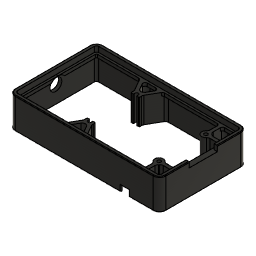
Apollo Vmount Body P3 [(P)MPLA000000170] v1 (Autodesk Fusion 360 design; units mm, degrees)
Autodesk Fusion 360 part; units mm, degrees
sketch "Sketch1" plane through (0, 0, 0) normal (0, 0, 1) x (1, 0, 0)
  line L0 (-70.75, 35.15) -> (-70.75, -35.15)
  arc A0 (-70.75, -35.15) -> (-64.75, -41.15) centre (-64.75, -35.15) ccw
  line L1 (-64.75, -41.15) -> (64.75, -41.15)
  arc A1 (64.75, -41.15) -> (70.75, -35.15) centre (64.75, -35.15) ccw
  line L2 (70.75, -35.15) -> (70.75, 35.15)
  arc A2 (70.75, 35.15) -> (64.75, 41.15) centre (64.75, 35.15) ccw
  line L3 (64.75, 41.15) -> (-64.75, 41.15)
  arc A3 (-64.75, 41.15) -> (-70.75, 35.15) centre (-64.75, 35.15) ccw
  circle A4 centre (-14, 22.05) radius 1.6
  circle A5 centre (51.15, -21.95) radius 4
  circle A6 centre (51.15, 22.05) radius 4
  line L4 (-14, -21.95) -> (70.75, -21.95)
  line L5 (-14, 41.15) -> (-14, -46.1385)
  line L6 (-14, 22.05) -> (87.0646, 22.05)
  circle A7 centre (-14, -21.95) radius 1.6
  line L7 (-15.5, 41.15) -> (-15.5, -46.1385)
  line L8 (-12.5, 41.15) -> (-12.5, -46.1385)
  line L9 (-65.75, -38.15) -> (65.75, -38.15)
  arc A8 (65.75, -38.15) -> (67.75, -36.15) centre (65.75, -36.15) ccw
  line L10 (67.75, -36.15) -> (67.75, 36.15)
  arc A9 (67.75, 36.15) -> (65.75, 38.15) centre (65.75, 36.15) ccw
  line L11 (65.75, 38.15) -> (-65.75, 38.15)
  arc A10 (-65.75, 38.15) -> (-67.75, 36.15) centre (-65.75, 36.15) ccw
  line L12 (-67.75, 36.15) -> (-67.75, -36.15)
  arc A11 (-67.75, -36.15) -> (-65.75, -38.15) centre (-65.75, -36.15) ccw
  line L13 (51.15, -41.15) -> (51.15, 41.15)
  line L14 (52.65, -41.15) -> (52.65, 41.15)
  line L15 (49.65, -41.15) -> (49.65, 41.15)
  line L16 (-14, -23.45) -> (70.75, -23.45)
  line L17 (-17.7081, -20.45) -> (70.75, -20.45)
  line L18 (-17.7081, 20.55) -> (87.0646, 20.55)
  line L19 (-14, 23.55) -> (87.0646, 23.55)
  circle A12 centre (-14, -21.95) radius 4
  circle A13 centre (-14, 22.05) radius 4
  line L20 (-15.5, 25.7581) -> (-22.6545, 38.15)
  line L21 (-15.5, -25.6581) -> (-22.7122, -38.15)
  line L22 (-17.7003, -23.4691) -> (-26.1763, -38.15)
  line L23 (-17.7003, 23.5691) -> (-26.1186, 38.15)
  line L24 (-12.5, 25.7581) -> (-5.3455, 38.15)
  line L25 (-12.5, -25.6581) -> (-5.2878, -38.15)
  line L26 (-10.3107, -23.45) -> (-1.8237, -38.15)
  line L27 (-10.2997, 23.5691) -> (-1.8814, 38.15)
  circle A14 centre (51.15, -21.95) radius 1.6
  circle A15 centre (51.15, 22.05) radius 1.6
  line L28 (-15, 41.15) -> (-15, -46.1385)
  line L29 (-13, 41.15) -> (-13, -46.1385)
  dimension "d49" = 3.2
  dimension "d50" = 8
  dimension "d51" = 8
  dimension "d52" = 6
  dimension "d53" = 82.3
  dimension "d54" = 41.15
  dimension "d55" = 141.5
  dimension "d56" = 70.75
  dimension "d57" = 3.2
  dimension "d58" = 19.6
  dimension "d59" = 19.2
  dimension "d60" = 65.15
  dimension "d61" = 44
  dimension "d62" = 1.5
  dimension "d63" = -1.5
  dimension "d65" = 1.5
  dimension "d66" = -1.5
  dimension "d67" = 1.5
  dimension "d71" = -1.5
  dimension "d72" = 8
  dimension "d73" = 8
  dimension "d74" = 60
  dimension "d75" = 60
  dimension "d78" = 3
  dimension "d79" = 3
  dimension "d80" = 60
  dimension "d81" = 60
  dimension "d84" = 3
  dimension "d85" = 3
  dimension "d86" = 3.2
  dimension "d87" = 3.2
  dimension "d107" = 1
  dimension "d108" = -1
  dimension "d111" = 2
  dimension "d112" = 2
  dimension "d113" = 6
  dimension "d114" = 6
  dimension "d115" = 6
  constraint horizontal L3
  constraint perpendicular L0 L3
  constraint parallel L1 L3
  constraint parallel L0 L2
  constraint tangent L3 A3
  constraint tangent L0 A3
  constraint tangent L0 A0
  constraint tangent A0 L1
  constraint tangent L1 A1
  constraint tangent A1 L2
  constraint tangent L2 A2
  constraint tangent A2 L3
  constraint perpendicular L1 L5
  constraint coincident A4.centre L6.start
  constraint perpendicular L2 L6
  constraint coincident L2 L4.end
  constraint coincident L3 L5.start
  constraint coincident L4.start L5
  constraint perpendicular L4 L5
  constraint coincident L4.start A7.centre
  constraint vertical A5.centre A6.centre
  constraint coincident A5.centre L4
  constraint vertical A4.centre L4.start
  constraint coincident A6.centre L6
  constraint coincident L1 L13.start
  constraint coincident L3 L13.end
  constraint coincident A5.centre L13
  constraint coincident A6.centre L13
  constraint concentric A7 A12
  constraint concentric A4 A13
  constraint coincident A13 L20.start
  constraint coincident L7 L20.start
  constraint coincident L11 L20.end
  constraint coincident A12 L21.start
  constraint coincident L7 L21.start
  constraint coincident L9 L21.end
  constraint parallel L21 L22
  constraint coincident A12 L22.start
  constraint coincident L9 L22.end
  constraint parallel L20 L23
  constraint coincident A13 L23.start
  constraint coincident L11 L23.end
  constraint coincident A13 L24.start
  constraint coincident L8 L24.start
  constraint coincident L11 L24.end
  constraint coincident A12 L25.start
  constraint coincident L9 L25.end
  constraint parallel L25 L26
  constraint coincident L9 L26.end
  constraint coincident L16 L26.start
  constraint parallel L24 L27
  constraint coincident A13 L27.start
  constraint coincident L11 L27.end
  constraint coincident L8 L25.start
  constraint concentric A5 A14
  constraint concentric A6 A15
  constraint parallel L4 L17
  constraint coincident A12 L17.start
  constraint parallel L6 L18
  constraint coincident A13 L18.start
  constraint parallel L1 L9
  constraint parallel L2 L10
  constraint parallel L3 L11
  constraint parallel L0 L12
  constraint tangent A9 L11
  constraint tangent L9 A11
  constraint tangent L9 A8
  constraint tangent A10 L12
  constraint tangent A8 L10
  constraint tangent L10 A9
  constraint tangent L12 A11
  constraint tangent L11 A10
  measures "d49" diameter of A4
  measures "d50" diameter of A6
  measures "d51" diameter of A5
  measures "d52" radius of A3
  measures "d53" distance of L1 L3
  measures "d54" distance of origin L1
  measures "d55" distance of L0 L2
  measures "d56" distance of origin L2
  measures "d57" diameter of A7
  measures "d58" distance of A5.centre L2
  measures "d59" distance of A5.centre L1
  measures "d60" distance of A5.centre L4.start
  measures "d61" distance of A5.centre A6.centre
  measures "d72" diameter of A12
  measures "d73" diameter of A13
  measures "d74" angle of L9 L21
  measures "d75" angle of L11 L20
  measures "d78" distance of L21 L22
  measures "d79" distance of L20 L23
  measures "d80" angle of L9 L25
  measures "d81" angle of L11 L24
  measures "d84" distance of L25 L26
  measures "d85" distance of L24 L27
  measures "d86" diameter of A14
  measures "d87" diameter of A15
  measures "d111" radius of A10
  measures "d112" radius of A11
  measures "d113" radius of A0
  measures "d114" radius of A1
  measures "d115" radius of A2
extrude "Extrude1" add sketch "Sketch1" along normal blind 29 contours L0 A0 L1 L3 A3 L7 L9 L11 A10 L12 A11 | L3 L7 L11 L28 | L1 L7 L9 L28 | L3 L5 L11 L28 | L1 L5 L9 L28 | L3 L5 L11 L29 | A4 L7 A13 L28 | A4 L7 L18 A13 | L11 A13 L20 L23 | L1 L5 L9 L29 | A7 L7 L17 A12 | L9 A12 L21 L22 | A7 L7 A12 L28 | L3 L8 L11 L29 | A4 L5 A13 L28 | L1 L8 L9 L29 | L5 A7 A12 L28 | L3 L8 L11 L15 | A4 L5 L19 A13 L29 | A4 L7 L18 L28 | L1 L8 L9 L15 | L5 A7 L16 A12 L29 | A7 L7 L17 L28 | L3 L11 L13 L15 | L8 L19 A13 L29 | L1 L9 L13 L15 | L8 L16 A12 L29 | L3 L11 L13 L14 | A6 L11 L13 L15 | L8 L19 A13 | L11 A13 L24 L27 | A4 L19 L29 | A4 L8 L19 L29 | L1 L9 L13 L14 | A5 L9 L13 L15 | L8 L16 A12 L26 | L9 A12 L25 L26 | A7 L8 L16 L29 | A7 L16 L29 | L2 A2 L3 L10 A9 L11 L14 L19 | A6 L11 L13 L14 | A6 L15 L19 | A6 L13 L15 L19 A15 | A4 L6 L8 L19 A13 | L1 A1 L2 L9 A8 L10 L14 L16 | A5 L9 L13 L14 | A5 L13 L15 L16 A14 | A5 L15 L16 | L4 A7 L8 L16 A12 | L16 A12 L26 | A6 L13 L14 L19 A15 | A6 L6 L15 L19 A15 | L15 L19 A15 | A5 L13 L14 L16 A14 | A5 L4 L15 L16 A14 | L15 L16 A14 | A6 L14 L19 | A6 L6 L15 L18 A15 | A4 L6 L8 L18 A13 | A4 L8 L18 L29 | A5 L14 L16 | A5 L4 L15 L17 A14 | L4 A7 L8 L17 A12 | A7 L8 L17 L29 | L2 L6 L10 L19 | A6 L6 L10 L19 | A6 L6 L14 L19 A15 | L14 L19 A15 | A6 L15 L18 | L2 L4 L10 L16 | A5 L4 L14 L16 A14 | A5 L4 L10 L16 | L14 L16 A14 | A5 L15 L17 | L2 L6 L10 L18 | A6 L6 L10 L18 | A6 L6 L14 L18 A15 | A6 L13 L15 L18 A15 | L15 L18 A15 | L2 L4 L10 L17 | A5 L4 L14 L17 A14 | A5 L4 L10 L17 | A5 L13 L15 L17 A14 | L15 L17 A14 | L2 L10 L17 L18 | A6 L14 L18 | A6 L13 L14 L18 A15 | A5 L14 L17 | A5 L13 L14 L17 A14 | L14 L18 A15 | L14 L17 A14
fillet "Fillet1" radius 3 32 edges at (-1.8237, -38.15, 14.5) (-22.7122, -38.15, 14.5) (-5.2878, -38.15, 14.5) (-26.1763, -38.15, 14.5) (-17.7003, -23.4691, 14.5) (-15.5, -25.6581, 14.5) (-12.5, -25.6581, 14.5) (54.8581, -20.45, 14.5) (54.8581, -23.45, 14.5) (52.65, -25.6581, 14.5) (49.65, -25.6581, 14.5) (52.65, -38.15, 14.5) (49.65, -38.15, 14.5) (67.75, -23.45, 14.5) (67.75, -20.45, 14.5) (-15.5, 25.7581, 14.5) (-12.5, 25.7581, 14.5) (-10.2997, 23.5691, 14.5) (-17.7003, 23.5691, 14.5) (-26.1186, 38.15, 14.5) (-22.6545, 38.15, 14.5) (-5.3455, 38.15, 14.5) (-1.8814, 38.15, 14.5) (49.65, 38.15, 14.5) (52.65, 38.15, 14.5) (52.65, 25.7581, 14.5) (54.8581, 23.55, 14.5) (49.65, 25.7581, 14.5) (67.75, 20.55, 14.5) (67.75, 23.55, 14.5) (54.8581, 20.55, 14.5) (-10.2997, -23.4691, 14.5)
sketch "Sketch2" plane through (0, 0, 29) normal (0, 0, 1) x (-1, 0, 0)
  arc A0 (-48.5786, -25.1139) -> (-54.2139, -19.4786) centre (-51.15, -22.05) ccw
  line L0 (-52.65, -27.4119) -> (-52.65, -35.15)
  line L1 (17.4583, -38.15) -> (10.5417, -38.15)
  arc A1 (-67.75, -36.15) -> (-65.75, -38.15) centre (-64.75, -35.15) ccw
  line L2 (-67.75, -17.55) -> (-67.75, 17.45)
  arc A2 (-65.75, 38.15) -> (-67.75, 36.15) centre (-64.75, 35.15) ccw
  line L3 (-65.75, 38.15) -> (-55.65, 38.15)
  line L4 (-52.65, 35.15) -> (-52.65, 27.3119)
  arc A3 (-54.2139, 19.3786) -> (-48.5786, 25.0139) centre (-51.15, 21.95) ccw
  line L5 (-49.65, 27.3119) -> (-49.65, 35.15)
  line L6 (-46.65, 38.15) -> (0.0916, 38.15)
  arc A4 (67.75, 36.15) -> (65.75, 38.15) centre (64.75, 35.15) ccw
  line L7 (67.75, 36.15) -> (67.75, -36.15)
  arc A5 (65.75, -38.15) -> (67.75, -36.15) centre (64.75, -35.15) ccw
  line L8 (65.75, -38.15) -> (27.8506, -38.15)
  line L9 (-49.65, -35.15) -> (-49.65, -27.4119)
  arc A6 (64.75, -41.15) -> (70.75, -35.15) centre (64.75, -35.15) ccw
  line L10 (70.75, -35.15) -> (70.75, 35.15)
  arc A7 (70.75, 35.15) -> (64.75, 41.15) centre (64.75, 35.15) ccw
  line L11 (64.75, 41.15) -> (-64.75, 41.15)
  arc A8 (-64.75, 41.15) -> (-70.75, 35.15) centre (-64.75, 35.15) ccw
  line L12 (-70.75, 35.15) -> (-70.75, -35.15)
  arc A9 (-70.75, -35.15) -> (-64.75, -41.15) centre (-64.75, -35.15) ccw
  line L13 (-64.75, -41.15) -> (64.75, -41.15)
  line L14 (25.2525, -36.65) -> (18.317, -24.6372)
  arc A10 (10.2919, -20.55) -> (10.0485, -22.6713) centre (14, -22.05) ccw
  line L15 (9.683, -24.6372) -> (2.7475, -36.65)
  line L16 (-64.75, -23.55) -> (-56.5119, -23.55)
  line L17 (13, -20.55) -> (10.2919, -20.55)
  line L18 (-64.75, 20.45) -> (-56.5119, 20.45)
  line L19 (-56.5119, 23.45) -> (-64.75, 23.45)
  line L20 (2.6897, 36.65) -> (9.683, 24.5372)
  arc A11 (10.0485, 22.5713) -> (10.2919, 20.45) centre (14, 21.95) ccw
  line L21 (18.317, 24.5372) -> (25.3103, 36.65)
  line L22 (20.1141, 33.65) -> (16.5981, 27.56)
  line L23 (11.4019, 27.56) -> (7.8859, 33.65)
  line L24 (16.5981, -27.66) -> (20.0564, -33.65)
  line L25 (7.9436, -33.65) -> (11.4019, -27.66)
  circle A12 centre (-51.15, 21.95) radius 1.6
  circle A13 centre (-51.15, -22.05) radius 1.6
  arc A14 (7.9436, -33.65) -> (10.5417, -38.15) centre (10.5417, -35.15) ccw
  arc A15 (16.5981, -27.66) -> (11.4019, -27.66) centre (14, -29.16) ccw
  arc A16 (17.4583, -38.15) -> (20.0564, -33.65) centre (17.4583, -35.15) ccw
  arc A17 (-49.65, 27.3119) -> (-48.5786, 25.0139) centre (-46.65, 27.3119) ccw
  arc A18 (-46.65, 38.15) -> (-49.65, 35.15) centre (-46.65, 35.15) ccw
  arc A19 (2.6897, 36.65) -> (0.0916, 38.15) centre (0.0916, 35.15) ccw
  arc A20 (18.317, 24.5372) -> (17.9515, 22.5713) centre (20.915, 23.0372) ccw
  arc A21 (27.9084, 38.15) -> (25.3103, 36.65) centre (27.9084, 35.15) ccw
  line L26 (27.9084, 38.15) -> (65.75, 38.15)
  arc A22 (25.2525, -36.65) -> (27.8506, -38.15) centre (27.8506, -35.15) ccw
  arc A23 (17.9515, -22.6713) -> (18.317, -24.6372) centre (20.915, -23.1372) ccw
  arc A24 (9.683, -24.6372) -> (10.0485, -22.6713) centre (7.085, -23.1372) ccw
  arc A25 (0.1494, -38.15) -> (2.7475, -36.65) centre (0.1494, -35.15) ccw
  line L27 (0.1494, -38.15) -> (-46.65, -38.15)
  arc A26 (-49.65, -35.15) -> (-46.65, -38.15) centre (-46.65, -35.15) ccw
  arc A27 (-48.5786, -25.1139) -> (-49.65, -27.4119) centre (-46.65, -27.4119) ccw
  arc A28 (-56.5119, -20.55) -> (-54.2139, -19.4786) centre (-56.5119, -17.55) ccw
  arc A29 (-67.75, -17.55) -> (-64.75, -20.55) centre (-64.75, -17.55) ccw
  arc A30 (-64.75, 20.45) -> (-67.75, 17.45) centre (-64.75, 17.45) ccw
  arc A31 (-54.2139, 19.3786) -> (-56.5119, 20.45) centre (-56.5119, 17.45) ccw
  arc A32 (-53.7214, 25.0139) -> (-52.65, 27.3119) centre (-55.65, 27.3119) ccw
  arc A33 (-53.7214, 25.0139) -> (-54.2139, 24.5214) centre (-51.15, 21.95) ccw
  arc A34 (-56.5119, 23.45) -> (-54.2139, 24.5214) centre (-56.5119, 26.45) ccw
  arc A35 (-67.75, 26.45) -> (-64.75, 23.45) centre (-64.75, 26.45) ccw
  line L28 (-67.75, 26.45) -> (-67.75, 36.15)
  arc A36 (-52.65, 35.15) -> (-55.65, 38.15) centre (-55.65, 35.15) ccw
  arc A37 (-55.65, -38.15) -> (-52.65, -35.15) centre (-55.65, -35.15) ccw
  line L29 (-55.65, -38.15) -> (-65.75, -38.15)
  line L30 (-67.75, -36.15) -> (-67.75, -26.55)
  arc A38 (-64.75, -23.55) -> (-67.75, -26.55) centre (-64.75, -26.55) ccw
  arc A39 (-54.2139, -24.6214) -> (-56.5119, -23.55) centre (-56.5119, -26.55) ccw
  arc A40 (-54.2139, -24.6214) -> (-53.7214, -25.1139) centre (-51.15, -22.05) ccw
  arc A41 (-52.65, -27.4119) -> (-53.7214, -25.1139) centre (-55.65, -27.4119) ccw
  arc A42 (11.4019, 27.56) -> (16.5981, 27.56) centre (14, 29.06) ccw
  arc A43 (10.0485, 22.5713) -> (9.683, 24.5372) centre (7.085, 23.0372) ccw
  line L31 (27.8506, -38.15) -> (-55.65, -38.15)
  line L32 (-67.75, -36.15) -> (-67.75, 26.45)
  line L33 (-55.65, 38.15) -> (27.9084, 38.15)
  line L34 (-67.75, 13.2) -> (-70.75, 13.2)
  line L35 (-67.75, -13.2) -> (-70.75, -13.2)
  arc A44 (13, -20.801) -> (15, -20.801) centre (14, -22.05) ccw
  line L36 (-56.5119, -20.55) -> (-64.75, -20.55)
  line L37 (10.2919, 20.45) -> (13, 20.45)
  arc A45 (15, 20.701) -> (13, 20.701) centre (14, 21.95) ccw
  arc A46 (17.7081, 20.45) -> (17.9515, 22.5713) centre (14, 21.95) ccw
  arc A47 (17.9515, -22.6713) -> (17.7081, -20.55) centre (14, -22.05) ccw
  line L38 (17.7081, -20.55) -> (15, -20.55)
  arc A48 (10.484, 38.15) -> (7.8859, 33.65) centre (10.484, 35.15) ccw
  line L39 (10.484, 38.15) -> (17.516, 38.15)
  arc A49 (20.1141, 33.65) -> (17.516, 38.15) centre (17.516, 35.15) ccw
  line L40 (13, 20.45) -> (13, 20.701)
  line L41 (15, 20.701) -> (15, 20.45)
  line L42 (15, 20.45) -> (17.7081, 20.45)
  line L43 (15, -20.55) -> (15, -20.801)
  line L44 (13, -20.801) -> (13, -20.55)
  line L45 (65.75, -35.15) -> (65.75, 35.15)
  arc A50 (65.75, 35.15) -> (64.75, 36.15) centre (64.75, 35.15) ccw
  line L46 (64.75, 36.15) -> (-64.75, 36.15)
  arc A51 (-64.75, 36.15) -> (-65.75, 35.15) centre (-64.75, 35.15) ccw
  line L47 (-65.75, 35.15) -> (-65.75, -35.15)
  arc A52 (-65.75, -35.15) -> (-64.75, -36.15) centre (-64.75, -35.15) ccw
  line L48 (-64.75, -36.15) -> (64.75, -36.15)
  arc A53 (64.75, -36.15) -> (65.75, -35.15) centre (64.75, -35.15) ccw
  point P0 (-64.75, 35.15)
  point P1 (-64.75, -35.15)
  point P2 (65.75, 36.15)
  point P3 (65.75, -36.15)
  point P4 (-64.75, 35.15)
  point P5 (-64.75, -35.15)
  point P6 (64.75, -35.15)
  point P7 (64.75, 35.15)
  point P8 (-65.75, 36.15)
  point P9 (-65.75, -36.15)
  point P10 (65.75, 36.15)
  point P11 (65.75, -36.15)
  dimension "d90" = -5
  dimension "d97" = 26.4
  dimension "d98" = 13.2
  constraint coincident L8.end A22.end
  constraint coincident A37.start L29.start
  constraint coincident A1.start L30.start
  constraint coincident A35.start L28.start
  constraint coincident L3.end A36.end
  constraint coincident A21.start L26.start
  constraint coincident L2 L34.start
  constraint coincident L12 L34.end
  constraint perpendicular L12 L34
  constraint coincident L2 L35.start
  constraint coincident L12 L35.end
  constraint perpendicular L12 L35
  measures "d97" distance of L34 L35
  measures "d98" distance of origin L34
extrude "Extrude2" cut sketch "Sketch2" against normal blind 5 contours A0 L0 L9 L16 A26 A27 A28 A29 A37 A38 A39 A40 A41 L36 L47 L48 | A0 A3 L5 L9 L14 A10 L15 L17 L18 L20 A11 L21 A17 A18 A20 A23 A24 A26 A27 A28 A29 A30 A31 A43 A44 L36 L37 A45 A46 A47 L38 L40 L41 L42 L43 L44 L45 A50 L46 L47 L48 A53 | A26 A37 L31 L48 | A29 A38 L32 L47 | L0 L16 A37 A38 A39 A40 A41 L47 A52 L48 | A1 A37 L29 L30 A38 L32 L47 A52 L48 | L15 A14 A25 L31 L48 | L14 A10 L15 L17 L24 L25 A14 A15 A16 A23 A24 A44 A47 L38 L43 L44 L48 | L4 A3 L5 L18 L19 A17 A18 A30 A31 A32 A33 A34 A35 A36 L46 L47 | A30 A35 L32 L47 | L1 A14 A16 L31 L48 | L24 L25 A14 A15 A16 L48 | L2 L12 L32 L34 L35 | L4 L19 A32 A33 A34 A35 A36 L46 A51 L47 | A2 L3 A35 L28 A36 L46 A51 L47 | L14 A16 A22 L31 L48 | A18 A36 L33 L46 | L6 L20 A18 A19 L33 L46 | L20 A11 L21 L22 L23 A20 A42 A43 L37 A45 A46 A48 A49 L40 L41 L42 L46 | L20 A19 L33 A48 L46 | L22 L23 A42 A48 A49 L46 | L21 A21 L33 A49 L46 | A12 | A13
extrude "Extrude5" add sketch "Sketch2" against normal blind 3 from surface at -5 contours L15 A25 L27 A26 L31 L48 | L2 A29 A30 L32 L47 | A1 A37 L29 L30 A38 L32 L47 A52 L48 | L1 A14 A16 L31 L48 | A2 L3 A35 L28 A36 L46 A51 L47 | A4 L7 A5 L8 L14 L21 A21 L26 A22 L45 A50 L46 L48 A53 | L6 L20 A18 A19 L33 L46 | L33 A48 L39 A49 L46 | L21 A21 L33 A49 L46
sketch "Sketch3" plane through (0, -41.15, 0) normal (0, -1, 0) x (1, 0, 0)
  line L0 (-66.4, 0) -> (66.4, 0)
  line L1 (66.4, 0) -> (66.4, 21)
  line L2 (-66.4, 21) -> (-66.4, 0)
  line L3 (33.8, 0) -> (42.4, 0)
  line L4 (42.4, 0) -> (42.4, 6.1)
  line L5 (42.4, 6.1) -> (33.8, 6.1)
  line L6 (33.8, 6.1) -> (33.8, 0)
  line L7 (32.1, 0) -> (44.1, 0)
  line L8 (44.1, 0) -> (44.1, 10)
  line L9 (44.1, 10) -> (32.1, 10)
  line L10 (32.1, 10) -> (32.1, 0)
  line L11 (66.4, 21) -> (-66.4, 21)
  line L12 (-64.75, 0) -> (64.75, 0)
  line L13 (64.75, 0) -> (64.75, 29)
  line L14 (-64.75, 29) -> (-64.75, 0)
  line L15 (64.75, 29) -> (-64.75, 29)
  line L16 (38.1, 6.1) -> (38.1, 10)
  circle A0 centre (-49.2, 16) radius 5.6
  circle A1 centre (-49.2, 16) radius 8
  dimension "d31" = 24
  dimension "d32" = 8.6
  dimension "d33" = 6.1
  dimension "d34" = 12
  dimension "d35" = 10
  dimension "d105" = 1.7
  dimension "d116" = 11.2
  dimension "d117" = 83
  dimension "d118" = 13
  dimension "d119" = 16
  constraint horizontal L3
  constraint vertical L4
  constraint horizontal L5
  constraint vertical L6
  constraint coincident L0 L3.start
  constraint horizontal L7
  constraint vertical L8
  constraint horizontal L9
  constraint vertical L10
  constraint coincident L0 L7.start
  constraint midpoint L5 L16.start
  constraint midpoint L9 L16.end
  constraint concentric A0 A1
  measures "d31" distance of L1 L4
  measures "d32" distance of L4 L6
  measures "d33" distance of L3 L5
  measures "d34" distance of L7.start L7.end
  measures "d35" distance of L7.start L9.end
  measures "d105" distance of L6 L10
  measures "d116" diameter of A0
  measures "d117" distance of L6 A0.centre
  measures "d118" distance of L15 A0.centre
  measures "d119" diameter of A1
extrude "Extrude3" cut sketch "Sketch3" along normal blind -1.8 and the other way blind 3 contours L0 L5 L6 L7 L9 L10 L12 L16 | L0 L4 L5 L7 L8 L9 L12 L16
extrude "Extrude4" cut sketch "Sketch3" against normal blind 3 contours L0 L3 L4 L5 L6 L7 L12
chamfer "Chamfer1" distance 0.6 angle 45 19 edges at (-70.75, 0, 29) (-70.75, 0, 29) (-68.9926, -39.3926, 29) (0, -41.15, 29) (68.9926, -39.3926, 29) (70.75, 24.175, 29) (70.75, -24.175, 29) (68.9926, 39.3926, 29) (0, 41.15, 29) (-68.9926, 39.3926, 29) (-15.475, -41.15, 0) (53.575, -41.15, 0) (68.9926, -39.3926, 0) (70.75, 0, 0) (68.9926, 39.3926, 0) (0, 41.15, 0) (-68.9926, 39.3926, 0) (-70.75, 0, 0) (-68.9926, -39.3926, 0)
fillet "Fillet2" radius 2 16 edges at (49.4784, -36.15, 22.5) (65.75, -20.2784, 22.5) (-2.9784, -36.15, 22.5) (52.8216, -36.15, 22.5) (65.75, -23.6216, 22.5) (65.75, 20.3784, 22.5) (49.4784, 36.15, 22.5) (-24.9639, 36.15, 22.5) (-7.7133, 36.15, 22.5) (-20.2867, 36.15, 22.5) (52.8216, 36.15, 22.5) (-3.0361, 36.15, 22.5) (65.75, 23.7216, 22.5) (-25.0216, -36.15, 22.5) (-7.6555, -36.15, 22.5) (-20.3445, -36.15, 22.5)
fillet "Fillet3" radius 0.5 12 edges at (-10.2919, -20.45, 12) (-17.7081, -20.45, 12) (-10.2919, 20.55, 12) (-17.7081, 20.55, 12) (-13, 20.55, 12) (-13, 20.801, 12) (-15, 20.55, 12) (-15, 20.801, 12) (-13, -20.45, 12) (-13, -20.701, 12) (-15, -20.45, 12) (-15, -20.701, 12)
sketch "Sketch5" plane through (-70.75, 0, 0) normal (-1, 0, 0) x (0, -1, 0)
  line L0 (-35.15, 0.6) -> (35.15, 0.6)
  line L1 (35.15, 0.6) -> (35.15, 28.4)
  line L2 (35.15, 28.4) -> (-35.15, 28.4)
  line L3 (-35.15, 28.4) -> (-35.15, 0.6)
  circle A0 centre (0, 16) radius 8
  circle A1 centre (0, 16) radius 5.6
  line L4 (35.15, 29) -> (-35.15, 29)
  dimension "d126" = 11.2
  dimension "d127" = 16
  dimension "d128" = 13
  constraint concentric A0 A1
  constraint vertical origin A0.centre
  measures "d126" diameter of A1
  measures "d127" diameter of A0
  measures "d128" distance of A0.centre L4
extrude "Extrude6" cut sketch "Sketch5" against normal blind 5 contours A1
extrude "Extrude7" cut sketch "Sketch5" along normal blind -3 and the other way blind 5 contours A0
equation "d7 = 8 mm"
equation "d29 = -1.00 mm - 4 mm"
equation "d50 = d7"
equation "d51 = d7"
equation "d54 = d53 / 2"
equation "d56 = d55 / 2"
equation "d98 = d97 / 2"
